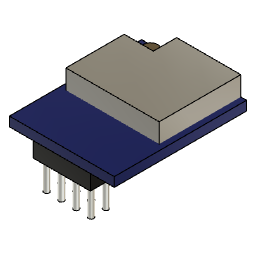
MLH2 v1.0 (Autodesk Fusion 360 archive; units mm, degrees)
design "RA-02"
Autodesk Fusion 360 part; units mm, degrees
sketch "Esquisse1" plane through (0, 0, 0) normal (0, 0, 1) x (1, 0, 0) in component "LoRa RA-02"
  line L0 (0, 0) -> (18, 0)
  line L1 (18, 0) -> (18, -22.7)
  line L2 (18, -22.7) -> (0, -22.7)
  line L3 (0, -22.7) -> (0, 0)
  line L4 (1, 0) -> (17, 0)
  line L5 (17, 0) -> (17, -14)
  line L6 (17, -14) -> (1, -14)
  line L7 (1, -14) -> (1, 0)
  line L8 (13.9, -22.7) -> (4.1, -22.7)
  line L9 (4.1, -22.7) -> (4.1, -17.7)
  line L10 (4.1, -17.7) -> (13.9, -17.7)
  line L11 (13.9, -17.7) -> (13.9, -22.7)
  line L12 (1, 0) -> (6, 0)
  line L13 (6, 0) -> (6, -4)
  line L14 (6, -4) -> (1, -4)
  line L15 (1, -4) -> (1, 0)
  circle A0 centre (3.5142, -2) radius 1.25
  circle A1 centre (5.2, -21.5) radius 0.445
  circle A2 centre (7.74, -21.5) radius 0.445
  circle A3 centre (10.28, -21.5) radius 0.445
  circle A4 centre (12.82, -21.5) radius 0.445
  circle A5 centre (5.2, -18.96) radius 0.445
  circle A6 centre (7.74, -18.96) radius 0.445
  circle A7 centre (10.28, -18.96) radius 0.445
  circle A8 centre (12.82, -18.96) radius 0.445
  dimension "d1" = 18
  dimension "d2" = 22.7
  dimension "d3" = 16
  dimension "d4" = 14
  dimension "d5" = 9.8
  dimension "d6" = 5
  dimension "d7" = 5
  dimension "d8" = 4
  dimension "d9" = 2.5
  dimension "d18" = 0.89
  dimension "d21" = 7.62
  dimension "d22" = 2.54
  dimension "d23" = 1.2
  dimension "d24" = 1.1
  constraint horizontal L0
  constraint vertical L1
  constraint horizontal L2
  constraint vertical L3
  constraint coincident L0.start L3.end
  constraint horizontal L4
  constraint vertical L5
  constraint horizontal L6
  constraint vertical L7
  constraint coincident L0 L4.start
  constraint midpoint L0 L4
  constraint horizontal L8
  constraint vertical L9
  constraint horizontal L10
  constraint vertical L11
  constraint coincident L2 L8.start
  constraint midpoint L2 L8
  constraint horizontal L12
  constraint vertical L13
  constraint horizontal L14
  constraint vertical L15
  measures "d1" distance of L0.start L0.end
  measures "d2" distance of L0.start L2.end
  measures "d3" distance of L4.start L4.end
  measures "d4" distance of L4.start L6.end
  measures "d5" distance of L8.start L8.end
  measures "d6" distance of L8.start L10.end
  measures "d7" distance of L4.start L12.end
  measures "d8" distance of L4.start L14.end
  measures "d9" diameter of A0
  measures "d18" diameter of A1
  measures "d23" distance of L2 A1.centre
  measures "d24" distance of L9 A1.centre
extrude "Extrusion1" add sketch "Esquisse1" along normal blind 1.6 contours L0 L1 L2 L3 L5 L6 L7 L9 L10 L11 L15 | L0 L4 L7 L12 L13 L14 L15 | L0 L4 L5 L6 L7 L13 L14 | L2 L8 L9 L10 L11 | A0 | A1 | A2 | A3 | A4 | A5 | A6 | A7 | A8 makes body 1 in component "LoRa RA-02"
extrude "Extrusion2" add sketch "Esquisse1" against normal blind 2.6 separate body contours L2 L8 L9 L10 L11 | A1 | A2 | A3 | A4 | A5 | A6 | A7 | A8 makes body 2 in component "LoRa RA-02"
extrude "Extrusion3" add sketch "Esquisse1" along normal blind 4.9 separate body contours L0 L4 L5 L6 L7 L13 L14 makes body 3 in component "LoRa RA-02"
extrude "Extrusion4" add sketch "Esquisse1" along normal blind 3 separate body contours A0 makes body 4 in component "LoRa RA-02"
extrude "Extrusion5" add sketch "Esquisse1" against normal blind 5 from surface at -2.6 separate body contours A1 | A2 | A3 | A4 | A5 | A6 | A7 | A8 makes body 5 at (10.077, -19.356, -4.2667) makes body 6 at (8.1712, -21.6098, -5.9333) makes body 7 at (12.617, -21.896, -4.2667) makes body 8 at (8.1712, -19.0698, -5.9333) makes body 9 at (12.617, -19.356, -4.2667) makes body 10 at (5.6312, -21.6098, -5.9333) makes body 11 at (10.077, -21.896, -4.2667) makes body 12 at (5.6312, -19.0698, -5.9333) in component "LoRa RA-02"
component "LoRa RA-02" placed x (1, 0, 0) y (0, 1, 0) z (0, 0, 1) at (0, 0, 0)
named bodies: "PCB", "connecteur", "SX11278", "IPX"

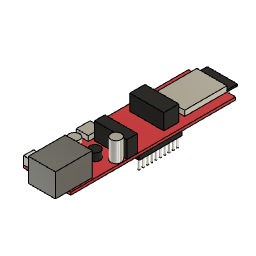
design "Olimex-POE-ISO"
Autodesk Fusion 360 part; units mm, degrees
sketch "Esquisse1" plane through (0, 0, 0) normal (0, 0, 1) x (1, 0, 0) in component "PCB"
sketch "Esquisse2" plane through (0, 0, 0) normal (0, 0, 1) x (1, 0, 0) in component "PCB"
  line L0 (-8, 49.5) -> (20.1, 49.5)
  line L1 (20.1, 49.5) -> (20.1, -48.9)
  line L2 (20.1, -48.9) -> (-8, -48.9)
  line L3 (-8, -48.9) -> (-8, 49.5)
  line L4 (-8, 17.5) -> (-5.5, 17.5)
  line L5 (-5.5, 17.5) -> (-5.5, -8)
  line L6 (-5.5, -8) -> (-8, -8)
  line L7 (-8, -8) -> (-8, 17.5)
  line L8 (20.1, 17.5) -> (17.4, 17.5)
  line L9 (17.4, 17.5) -> (17.4, -8.1)
  line L10 (17.4, -8.1) -> (20.1, -8.1)
  line L11 (20.1, -8.1) -> (20.1, 17.5)
  circle A0 centre (18.71, -6.7364) radius 0.5
  circle A1 centre (-6.69, -6.7364) radius 0.5
  circle A2 centre (18.71, -4.1964) radius 0.5
  circle A3 centre (-6.69, -4.1964) radius 0.5
  circle A4 centre (18.71, -1.6564) radius 0.5
  circle A5 centre (-6.69, -1.6564) radius 0.5
  circle A6 centre (18.71, 0.8836) radius 0.5
  circle A7 centre (-6.69, 0.8836) radius 0.5
  circle A8 centre (18.71, 3.4236) radius 0.5
  circle A9 centre (-6.69, 3.4236) radius 0.5
  circle A10 centre (18.71, 5.9636) radius 0.5
  circle A11 centre (-6.69, 5.9636) radius 0.5
  circle A12 centre (18.71, 8.5036) radius 0.5
  circle A13 centre (-6.69, 8.5036) radius 0.5
  circle A14 centre (18.71, 11.0436) radius 0.5
  circle A15 centre (-6.69, 11.0436) radius 0.5
  circle A16 centre (18.71, 13.5836) radius 0.5
  circle A17 centre (-6.69, 13.5836) radius 0.5
  circle A18 centre (18.71, 16.1236) radius 0.5
  circle A19 centre (-6.69, 16.1236) radius 0.5
  dimension "d27" = 1
  dimension "d30" = -25.4
  dimension "d31" = 22.86
  constraint horizontal L0
  constraint vertical L1
  constraint horizontal L2
  constraint vertical L3
  constraint horizontal L4
  constraint vertical L5
  constraint horizontal L6
  constraint vertical L7
  constraint coincident L3 L4.start
  constraint horizontal L8
  constraint vertical L9
  constraint horizontal L10
  constraint vertical L11
  constraint coincident L1 L8.start
  measures "d27" diameter of A0
extrude "Extrusion1" add sketch "Esquisse2" along normal blind 1.6 contours L0 L1 L2 L3 L4 L5 L6 L8 L9 L10 | L3 L4 L5 L6 L7 | L1 L8 L9 L10 L11 | A0 | A1 | A2 | A3 | A4 | A5 | A6 | A7 | A8 | A9 | A10 | A11 | A12 | A13 | A14 | A15 | A16 | A17 | A18 | A19 makes body 1 in component "PCB"
sketch "Esquisse3" plane through (0, 0, 1.6) normal (0, 0, 1) x (-1, 0, 0) in component "PCB"
  line L0 (8, 48.9) -> (-20.1, 48.9)
  line L1 (-20.1, 48.9) -> (-20.1, -49.5)
  line L2 (-20.1, -49.5) -> (8, -49.5)
  line L3 (8, -49.5) -> (8, 48.9)
  line L4 (-3, 35) -> (-19.1, 35)
  line L5 (-19.1, 35) -> (-19.1, 57)
  line L6 (-19.1, 57) -> (-3, 57)
  line L7 (-3, 57) -> (-3, 35)
  line L8 (3, -24.2) -> (-15, -24.2)
  line L9 (-15, -24.2) -> (-15, -55.7)
  line L10 (-15, -55.7) -> (3, -55.7)
  line L11 (3, -55.7) -> (3, -24.2)
  line L12 (4, -19.5) -> (-16.2318, -19.5)
  line L13 (-16.2318, -19.5) -> (-16.2318, -10.5189)
  line L14 (-16.2318, -10.5189) -> (4, -10.5189)
  line L15 (4, -10.5189) -> (4, -19.5)
  line L16 (8, 17.5) -> (0.8, 17.5)
  line L17 (0.8, 17.5) -> (0.8, 9.25)
  line L18 (0.8, 9.25) -> (8, 9.25)
  line L19 (8, 9.25) -> (8, 17.5)
  line L20 (-0.5554, 15.2069) -> (-20, 15.2069)
  line L21 (-20, 15.2069) -> (-20, 9)
  line L22 (-20, 9) -> (-0.5554, 9)
  line L23 (-0.5554, 9) -> (-0.5554, 15.2069)
  circle A0 centre (-16.8, 18.5) radius 3.1064
  circle A1 centre (-4.5, 31.1) radius 3.1064
  circle A2 centre (-9.4535, 23.7397) radius 3.0869
  line L24 (8, 48.9) -> (2, 48.9)
  line L25 (2, 48.9) -> (2, 42.9)
  line L26 (2, 42.9) -> (8, 42.9)
  line L27 (8, 42.9) -> (8, 48.9)
  dimension "d5" = 7.2
  dimension "d6" = 8.25
  dimension "d7" = 6
  dimension "d8" = 6
  constraint horizontal L4
  constraint vertical L5
  constraint horizontal L6
  constraint vertical L7
  constraint horizontal L8
  constraint vertical L9
  constraint horizontal L10
  constraint vertical L11
  constraint horizontal L12
  constraint vertical L13
  constraint horizontal L14
  constraint vertical L15
  constraint horizontal L16
  constraint vertical L17
  constraint horizontal L18
  constraint vertical L19
  constraint coincident L3 L16.start
  constraint horizontal L20
  constraint vertical L21
  constraint horizontal L22
  constraint vertical L23
  constraint horizontal L24
  constraint vertical L25
  constraint horizontal L26
  constraint vertical L27
  constraint coincident L0.start L3.end
  measures "d5" distance of L16.start L16.end
  measures "d6" distance of L16.start L18.end
  measures "d7" distance of L0.start L24.end
  measures "d8" distance of L0.start L26.end
extrude "Extrusion2" add sketch "Esquisse3" along normal blind 14 separate body contours L0 L4 L5 L7 | L0 L5 L6 L7 makes body 2 in component "PCB"
extrude "Extrusion3" add sketch "Esquisse3" along normal blind 4.8 separate body contours L0 L3 L24 L25 L26 L27 makes body 3 in component "PCB"
extrude "Extrusion4" add sketch "Esquisse3" along normal blind 3 separate body contours L3 L16 L17 L18 L19 makes body 4 in component "PCB"
extrude "Extrusion5" add sketch "Esquisse3" along normal blind 3.2 separate body contours L2 L8 L9 L11 makes body 5 in component "PCB"
extrude "Extrusion6" add sketch "Esquisse3" along normal blind 1 separate body contours L2 L9 L10 L11 makes body 6 in component "PCB"
extrude "Extrusion7" add sketch "Esquisse3" along normal blind 9.4 separate body contours L12 L13 L14 L15 makes body 7 in component "PCB"
extrude "Extrusion8" add sketch "Esquisse3" along normal blind 11.9 separate body contours A0 | A1 makes body 8 at (13.6974, -18.3452, 9.5333) makes body 9 at (1.3974, -30.9452, 9.5333) in component "PCB"
extrude "Extrusion9" add sketch "Esquisse3" along normal blind 4.5 separate body contours A2 makes body 10 in component "PCB"
extrude "Extrusion10" add sketch "Esquisse3" along normal blind 10.2 separate body contours L20 L21 L22 L23 makes body 11 in component "PCB"
extrude "Extrusion11" add sketch "Esquisse2" against normal blind 2.45 separate body contours L3 L4 L5 L6 L7 | L1 L8 L9 L10 L11 | A0 | A1 | A2 | A3 | A4 | A5 | A6 | A7 | A8 | A9 | A10 | A11 | A12 | A13 | A14 | A15 | A16 | A17 | A18 | A19 makes body 12 at (18.3, 8.9667, 0) makes body 13 at (-7.1667, 0.5, 0) in component "PCB"
extrude "Extrusion12" add sketch "Esquisse2" against normal blind 6 from surface at -2.45 separate body contours A0 | A1 | A2 | A3 | A4 | A5 | A6 | A7 | A8 | A9 | A10 | A11 | A12 | A13 | A14 | A15 | A16 | A17 | A18 | A19 makes body 14 at (-6.1906, -1.6814, -6.45) makes body 15 at (-6.1906, 8.4786, -6.45) makes body 16 at (19.1707, 16.3178, -6.45) makes body 17 at (18.3792, 5.5887, -6.45) makes body 18 at (18.3792, -4.5713, -6.45) makes body 19 at (18.3609, -1.2985, -6.45) makes body 20 at (19.0408, 8.8784, -6.45) makes body 21 at (-6.2293, 16.3178, -6.45) makes body 22 at (-6.1906, 5.9386, -6.45) makes body 23 at (-6.1906, -4.2214, -6.45) makes body 24 at (-6.1906, 0.8586, -6.45) makes body 25 at (-6.1906, 11.0186, -6.45) makes body 26 at (19.0408, 13.9584, -6.45) makes body 27 at (19.0408, 3.7984, -6.45) makes body 28 at (18.3792, -7.1113, -6.45) makes body 29 at (18.3609, 1.2415, -6.45) makes body 30 at (19.0408, 11.4184, -6.45) makes body 31 at (-6.1906, 13.5586, -6.45) makes body 32 at (-6.1906, 3.3986, -6.45) makes body 33 at (-6.1906, -6.7614, -6.45) in component "PCB"
component "PCB" placed x (1, 0, 0) y (0, 1, 0) z (0, 0, 1) at (0, 0, 0)
named bodies: "PCB", "RJ45", "JST", "USB", "ESP WROOM", "Antenna", "Connector", "C26", "C27", "L4", "DCDC", "EXT1"
